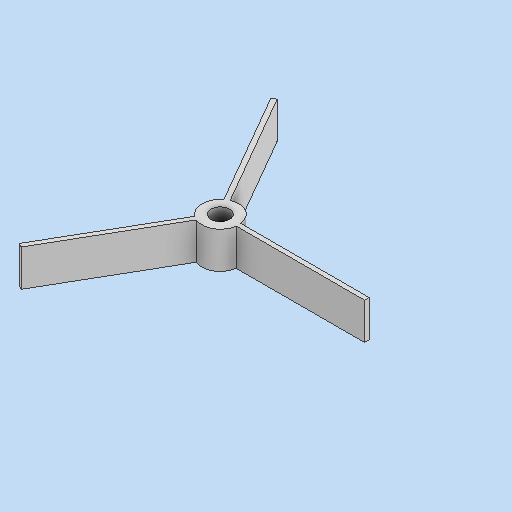
# Autodesk Inventor part: brush_tpu_test_print
Saved by Autodesk Inventor 2026 (Build 300175000, 175)
## iProperties
Created: 2026-02-09
Part Number: brush_tpu_test_print
Material: Generic
Document SubType Name: Modeling
Designer: mones
Density: 1 g/cm^3
Appearance: Default
Author: mones
Autodesk Inventor part; units mm, degrees
ref_plane "YZ Plane" through (0, 0, 0) normal (1, 0, 0) x (0, 1, 0)
ref_plane "XZ Plane" through (0, 0, 0) normal (0, 1, 0) x (-1, 0, 0)
ref_plane "XY Plane" through (0, 0, 0) normal (0, 0, 1) x (1, 0, 0)
sketch "Sketch1" plane through (0, 0, 0) normal (0, 1, 0) x (-1, 0, 0)
  circle A0 centre (0, 0) radius 6.35
  circle A1 centre (0, 0) radius 3.175
  line L0 (0, 0) -> (-25.4, 0)
  line L1 (0, 0) -> (12.7, -21.997)
  line L2 (0, 0) -> (12.7, 21.997)
  line L3 (12.0126, 22.3939) -> (13.3874, 21.6002)
  line L4 (13.3874, 21.6002) -> (-0.6874, 0.3969) construction
  line L5 (0.6874, -0.3969) -> (12.0126, 22.3939) construction
  line L6 (0, -0.7937) -> (0, 0)
  line L7 (0, 0.7937) -> (-25.4, -0.7937) construction
  line L8 (-25.4, 0.7937) -> (0, -0.7937) construction
  line L9 (0.6874, 0.3969) -> (12.0126, -22.3939) construction
  line L10 (13.3874, -21.6002) -> (-0.6874, -0.3969) construction
  line L11 (-25.4, -0.7937) -> (-3.0742, -0.7937)
  line L12 (-3.0742, 0.7937) -> (-25.4, 0.7937)
  line L13 (0.8497, 3.0592) -> (12.0126, 22.3939)
  line L14 (13.3874, 21.6002) -> (2.2245, 2.2654)
  line L15 (2.2245, -2.2654) -> (13.3874, -21.6002)
  line L16 (12.0126, -22.3939) -> (0.8497, -3.0592)
  line L17 (-25.4, 0) -> (-50.8, 0)
  line L18 (12.7, -21.997) -> (25.4, -43.9941)
  line L19 (12.7, 21.997) -> (25.4, 43.9941)
  line L20 (26.0874, 43.5972) -> (13.3874, 21.6002)
  line L21 (13.3874, 21.6002) -> (12.0126, 22.3939)
  line L22 (12.0126, 22.3939) -> (24.7126, 44.391)
  line L23 (24.7126, 44.391) -> (26.0874, 43.5972)
  line L24 (26.0874, 43.5972) -> (12.0126, 22.3939) construction
  line L25 (13.3874, 21.6002) -> (24.7126, 44.391) construction
  line L26 (26.0627, -43.5544) -> (12.0373, -22.4367) construction
  line L27 (13.4121, -21.643) -> (24.6879, -44.3482) construction
  line L28 (-50.8, 0.7937) -> (-25.4, 0.7937)
  line L29 (-25.4, -0.7937) -> (-50.8, -0.7937)
  line L30 (-50.8, -0.7937) -> (-50.8, 0.7937)
  line L31 (-50.8, 0.7937) -> (-25.4, -0.7937) construction
  line L32 (-25.4, 0.7937) -> (-50.8, -0.7937) construction
  line L33 (24.7126, -44.391) -> (12.0126, -22.3939)
  line L34 (13.3874, -21.6002) -> (26.0874, -43.5972)
  line L35 (26.0874, -43.5972) -> (24.7126, -44.391)
  line L36 (24.7126, -44.391) -> (13.3874, -21.6002) construction
  line L37 (12.0126, -22.3939) -> (26.0874, -43.5972) construction
  point P0 (6.35, 10.9985)
  point P1 (-12.7, 0)
  point P2 (6.35, -10.9985)
  point P3 (3.8375, -5.0593)
  point P4 (3.175, -5.4993)
  point P5 (-6.3002, -0.7937)
  point P6 (2.4627, -5.853)
  point P7 (3.8375, 5.0593)
  point P8 (2.4627, 5.853)
  point P9 (-6.3002, 0.7938)
  point P10 (19.05, 32.9956)
  point P11 (19.05, -32.9956)
  point P12 (-38.1, 0)
  constraints: 76 end point, 20 midpoint, 12 parallel, 6 point on circle, 2 centre point, 2 horizontal, 1 coincident, 1 perpendicular, 7 other
extrude "Extrusion1" add sketch "Sketch1" along normal blind 12.7 contours A0 L15 A1 L14 | L14 A1 L2 A0 | A0 L2 L3 L14 | L15 L34 L35 L18 L1 A0 | A0 L1 A1 L15 | L2 A1 L13 A0 | A0 L13 L3 L2 | L3 L19 L23 L20 | L1 L18 L35 L33 L16 A0 | A0 L16 A1 L1 | L13 A1 L12 A0 | L3 L22 L23 L19 | A0 L11 A1 L16 | L12 A1 L0 A0 | A0 L0 L17 L30 L28 L12 | L11 L29 L30 L17 L0 A0 | A0 L0 A1 L11
body "Solid1"
